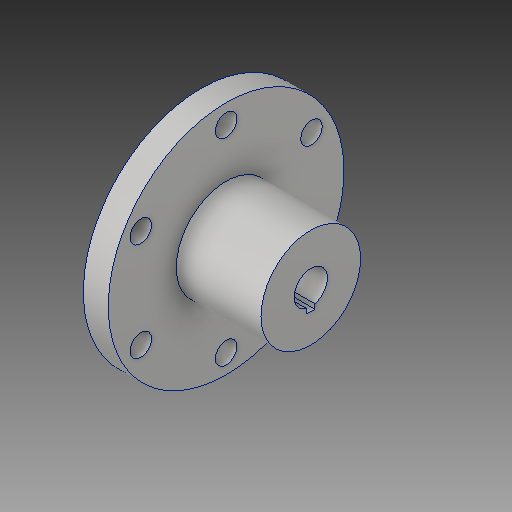
# Autodesk Inventor part: 10mmkethub18025
Saved by Autodesk Inventor 2019 (Build 230136000, 136)
## iProperties
Created: 2018-09-03
Part Number: 10mmkethub18025
Material: 一般
Document SubType Name: Modeling
Designer: シュンダイ
Density: 1 g/cm^3
Appearance: アルミニウム - フラット
Author: シュンダイ
Autodesk Inventor part; units mm, degrees
ref_plane "YZ Plane" through (0, 0, 0) normal (1, 0, 0) x (0, 1, 0)
ref_plane "XZ Plane" through (0, 0, 0) normal (0, 1, 0) x (-1, 0, 0)
ref_plane "XY Plane" through (0, 0, 0) normal (0, 0, 1) x (1, 0, 0)
sketch "スケッチ1" plane through (0, 0, 0) normal (1, 0, 0) x (0, 1, 0)
  point P0 (0, 0)
sketch "スケッチ2" plane through (0, 0, 0) normal (1, 0, 0) x (0, 1, 0)
  circle A0 centre (0, 0) radius 28.4
  dimension "d0" = 56.8
  constraints: 1 centre point, 1 coincident
  measures "d0" diameter of A0
extrude "押し出し1" add sketch "スケッチ2" along normal blind 6
sketch "スケッチ3" plane through (6, 0, 0) normal (1, 0, 0) x (0, 0, -1)
  circle A0 centre (0, 0) radius 12
  dimension "d3" = 24
  constraints: 1 centre point, 1 coincident
  measures "d3" diameter of A0
extrude "押し出し2" add sketch "スケッチ3" along normal blind 20.4
hole "穴2" at (26.4, 0, 0) direction (-1, 0, 0) diameter 8 end through all
sketch "スケッチ6" plane through (26.4, 0, 0) normal (1, 0, 0) x (0, 0, -1)
  line L0 (0, -5) -> (-1, -5)
  line L1 (-1, -5) -> (-1, -3)
  line L2 (-1, -5) -> (1, -5) construction
  line L3 (-1, -3) -> (1, -3)
  line L4 (1, -3) -> (1, -5)
  line L5 (1, -5) -> (0, -5)
  point P0 (0, 0)
  dimension "d32" = 5
  dimension "d33" = 1
  dimension "d35" = 2
  dimension "d36" = 90
  dimension "d37" = 2
  dimension "d38" = 90
  dimension "d39" = 2
  dimension "d40" = 90
  constraints: 12 end point, 3 perpendicular, 1 horizontal, 1 vertical
  measures "d32" distance of point (0, 0) L0.start
  measures "d33" distance of L0.start L0.end
  measures "d35" distance of L0.end L1.end
  measures "d36" angle of L2 L1
  measures "d37" distance of L1.end L3.end
  measures "d38" angle of L1 L3
  measures "d39" distance of L3.end L4.end
  measures "d40" angle of L3 L4
extrude "押し出し5" cut sketch "スケッチ6" against normal blind 26.4
sketch "スケッチ7" plane through (0, 0, 0) normal (-1, 0, 0) x (0, 0, 1)
  circle A0 centre (0, 0) radius 23.75
  line L0 (0, -23.75) -> (-20.5681, -11.875)
  line L1 (-20.5681, -11.875) -> (-20.5681, 11.875)
  line L2 (-20.5681, 11.875) -> (0, 23.75)
  line L3 (0, 23.75) -> (20.5681, 11.875)
  line L4 (20.5681, 11.875) -> (20.5681, -11.875)
  line L5 (20.5681, -11.875) -> (0, -23.75)
  dimension "d43" = 47.5
  constraints: 12 end point, 2 coincident, 1 vertical alignment, 15 other
hole "穴3" at (0, 11.875, 20.5681) at (0, 23.75, 0) at (0, -11.875, 20.5681) at (0, -23.75, 0) at (0, -11.875, -20.5681) at (0, 11.875, -20.5681) direction (1, 0, 0) diameter 5.2 end through all
